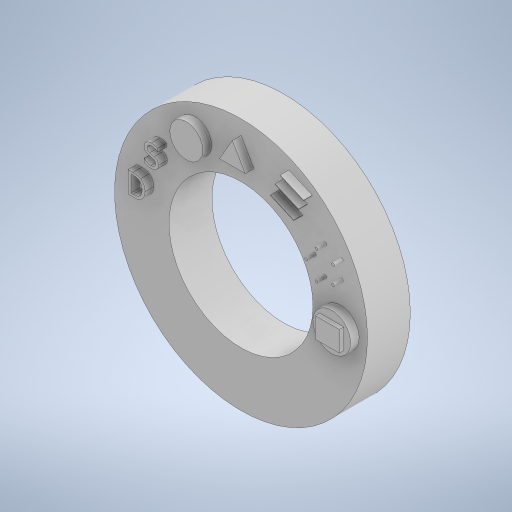
# Autodesk Inventor part: lab5CADfiguras
Saved by Autodesk Inventor 2023 (Build 270158000, 158)
## iProperties
Created: 2022-10-28
Part Number: lab5CADfiguras
Material: Generic
Document SubType Name: Modeling
Designer: jhair
Density: 1 g/cm^3
Appearance: Default
Author: jhair
Autodesk Inventor part; units mm, degrees
ref_plane "YZ Plane" through (0, 0, 0) normal (1, 0, 0) x (0, 1, 0)
ref_plane "XZ Plane" through (0, 0, 0) normal (0, 1, 0) x (-1, 0, 0)
ref_plane "XY Plane" through (0, 0, 0) normal (0, 0, 1) x (1, 0, 0)
sketch "Sketch1" plane through (0, 0, 0) normal (0, 0, 1) x (1, 0, 0)
  circle A0 centre (0, 0) radius 295
  circle A1 centre (0, 0) radius 168
  dimension "d0" = 590
  dimension "d1" = 336
  constraints: 2 centre point, 2 coincident
  measures "d0" diameter of A0
  measures "d1" diameter of A1
extrude "Extrusion1" add sketch "Sketch1" along normal blind 100
sketch "Sketch2" plane through (0, 0, 100) normal (0, 0, 1) x (1, 0, 0)
  line L0 (-208.7862, 161.4608) -> (-164.9221, 161.4608) construction
  line L1 (-164.9221, 161.4608) -> (-164.9221, 101.3592) construction
  line L2 (-164.9221, 101.3592) -> (-208.7862, 101.3592) construction
  line L3 (-208.7862, 101.3592) -> (-208.7862, 161.4608) construction
  line L4 (-248.2148, 80.7284) -> (-204.3506, 80.7284) construction
  line L5 (-204.3506, 80.7284) -> (-204.3506, 20.6268) construction
  line L6 (-204.3506, 20.6268) -> (-248.2148, 20.6268) construction
  line L7 (-248.2148, 20.6268) -> (-248.2148, 80.7284) construction
  spline S0 degree 2 poles (-189.783, 109.678) (-195.2125, 109.678) (-202.83, 111.947) (-206.193, 113.5678) knots 0 0 0 1 2 2 2
  line L8 (-206.193, 113.5678) -> (-206.193, 121.9146)
  line L9 (-206.193, 121.9146) -> (-205.7068, 121.9146)
  spline S1 degree 2 poles (-205.7068, 121.9146) (-202.4248, 118.8352) (-194.1185, 115.4316) (-190.2692, 115.4316) knots 0 0 0 1 2 2 2
  spline S2 degree 2 poles (-190.2692, 115.4316) (-184.7587, 115.4316) (-179.1266, 120.0102) (-179.1266, 123.7785) knots 0 0 0 1 2 2 2
  spline S3 degree 2 poles (-179.1266, 123.7785) (-179.1266, 126.7768) (-182.0845, 130.5046) (-185.2854, 131.4365) knots 0 0 0 1 2 2 2
  spline S4 degree 2 poles (-185.2854, 131.4365) (-187.595, 132.0848) (-191.4443, 132.9762) (-194.3211, 133.7055) knots 0 0 0 1 2 2 2
  spline S5 degree 2 poles (-194.3211, 133.7055) (-196.9143, 134.3943) (-201.0067, 136.4608) (-202.5869, 138.1221) knots 0 0 0 1 2 2 2
  spline S6 degree 2 poles (-202.5869, 138.1221) (-204.1266, 139.7833) (-205.8284, 144.2404) (-205.8284, 147.1577) knots 0 0 0 1 2 2 2
  spline S7 degree 2 poles (-205.8284, 147.1577) (-205.8284, 153.2355) (-196.347, 161.4608) (-189.0131, 161.4608) knots 0 0 0 1 2 2 2
  spline S8 degree 2 poles (-189.0131, 161.4608) (-184.7992, 161.4608) (-177.3438, 159.7995) (-174.1428, 158.2193) knots 0 0 0 1 2 2 2
  line L10 (-174.1428, 158.2193) -> (-174.1428, 150.2776)
  line L11 (-174.1428, 150.2776) -> (-174.629, 150.2776)
  spline S9 degree 2 poles (-174.629, 150.2776) (-177.0196, 152.4657) (-184.4751, 155.7071) (-188.5674, 155.7071) knots 0 0 0 1 2 2 2
  spline S10 degree 2 poles (-188.5674, 155.7071) (-193.1866, 155.7071) (-198.8997, 151.3717) (-198.8997, 147.8465) knots 0 0 0 1 2 2 2
  spline S11 degree 2 poles (-198.8997, 147.8465) (-198.8997, 144.6861) (-195.5366, 140.9178) (-192.3762, 140.067) knots 0 0 0 1 2 2 2
  spline S12 degree 2 poles (-192.3762, 140.067) (-190.2692, 139.4997) (-184.1509, 138.041) (-182.125, 137.4332) knots 0 0 0 1 2 2 2
  spline S13 degree 2 poles (-182.125, 137.4332) (-176.9791, 135.853) (-172.1979, 129.4916) (-172.1979, 124.8319) knots 0 0 0 1 2 2 2
  spline S14 degree 2 poles (-172.1979, 124.8319) (-172.1979, 121.8741) (-174.5885, 116.2015) (-176.736, 114.2161) knots 0 0 0 1 2 2 2
  spline S15 degree 2 poles (-176.736, 114.2161) (-179.1266, 112.0281) (-185.2044, 109.678) (-189.783, 109.678) knots 0 0 0 1 2 2 2
  spline S16 degree 2 poles (-203.7253, 55.6879) (-203.7253, 48.8402) (-209.2764, 37.8192) (-213.936, 34.7397) knots 0 0 0 1 2 2 2
  spline S17 degree 2 poles (-213.936, 34.7397) (-217.7448, 32.3491) (-225.5648, 30.7284) (-231.6426, 30.7284) knots 0 0 0 1 2 2 2
  line L12 (-231.6426, 30.7284) -> (-243.1499, 30.7284)
  line L13 (-243.1499, 30.7284) -> (-243.1499, 80.7284)
  line L14 (-243.1499, 80.7284) -> (-231.7642, 80.7284)
  spline S18 degree 2 poles (-231.7642, 80.7284) (-224.714, 80.7284) (-216.6913, 78.6214) (-213.855, 76.7576) knots 0 0 0 1 2 2 2
  spline S19 degree 2 poles (-213.855, 76.7576) (-209.0332, 73.5566) (-203.7253, 62.9812) (-203.7253, 55.6879) knots 0 0 0 1 2 2 2
  spline S20 degree 2 poles (-210.654, 55.7689) (-210.654, 61.5226) (-214.4627, 69.6668) (-218.231, 71.9764) knots 0 0 0 1 2 2 2
  spline S21 degree 2 poles (-218.231, 71.9764) (-220.9052, 73.5566) (-226.9425, 74.9748) (-231.4401, 74.9748) knots 0 0 0 1 2 2 2
  line L15 (-231.4401, 74.9748) -> (-236.5049, 74.9748)
  line L16 (-236.5049, 74.9748) -> (-236.5049, 36.482)
  line L17 (-236.5049, 36.482) -> (-231.4401, 36.482)
  spline S22 degree 2 poles (-231.4401, 36.482) (-227.0235, 36.482) (-220.3379, 37.9002) (-217.6232, 39.8046) knots 0 0 0 1 2 2 2
  spline S23 degree 2 poles (-217.6232, 39.8046) (-214.1386, 42.1547) (-210.654, 49.9342) (-210.654, 55.7689) knots 0 0 0 1 2 2 2
  point P0 (0, 0)
  constraints: 4 other
extrude "Extrusion2" add sketch "Sketch2" along normal blind 20
sketch "Sketch3" plane through (0, 0, 100) normal (0, 0, 1) x (1, 0, 0)
  circle A0 centre (-107.4544, 206.725) radius 38.7006
  line L0 (0, 260.9541) -> (30, 208.9926)
  line L1 (0, 260.9541) -> (60, 260.9541) construction
  line L2 (30, 208.9926) -> (-30, 208.9926)
  line L3 (-30, 208.9926) -> (0, 260.9541)
  line L4 (99.1241, 221.6176) -> (153.8823, 198.1595)
  line L5 (153.8823, 198.1595) -> (154.5516, 199.7218)
  line L6 (154.5516, 199.7218) -> (99.7934, 223.1799)
  line L7 (99.7934, 223.1799) -> (99.1241, 221.6176)
  line L8 (99.1241, 221.6176) -> (154.5516, 199.7218) construction
  line L9 (153.8823, 198.1595) -> (99.7934, 223.1799) construction
  line L10 (88.1405, 193.8335) -> (142.8987, 170.3754)
  line L11 (142.8987, 170.3754) -> (143.568, 171.9378)
  line L12 (143.568, 171.9378) -> (88.8098, 195.3958)
  line L13 (88.8098, 195.3958) -> (88.1405, 193.8335)
  line L14 (88.1405, 193.8335) -> (143.568, 171.9378) construction
  line L15 (142.8987, 170.3754) -> (88.8098, 195.3958) construction
  line L16 (110.8556, 245.3816) -> (165.6138, 221.9235)
  line L17 (165.6138, 221.9235) -> (166.2831, 223.4858)
  line L18 (166.2831, 223.4858) -> (111.5249, 246.9439)
  line L19 (111.5249, 246.9439) -> (110.8556, 245.3816)
  circle A1 centre (206.6962, 106.977) radius 34.8144
  circle A2 centre (171.8818, 106.977) radius 3.4311
  circle A3 centre (195.938, 73.8666) radius 3.4311
  circle A4 centre (234.8616, 86.5136) radius 3.4311
  circle A5 centre (234.8616, 127.4404) radius 3.4311
  circle A6 centre (195.938, 140.0875) radius 3.4311
  circle A7 centre (231.7388, -10.0458) radius 44.0014
  line L20 (199.303, 19.687) -> (264.1746, 19.687)
  line L21 (264.1746, 19.687) -> (264.1746, -39.7787)
  line L22 (264.1746, -39.7787) -> (199.303, -39.7787)
  line L23 (199.303, -39.7787) -> (199.303, 19.687)
  line L24 (199.303, 19.687) -> (264.1746, -39.7787) construction
  line L25 (264.1746, 19.687) -> (199.303, -39.7787) construction
  point P0 (0, 0)
  point P1 (126.8379, 210.6697)
  point P2 (115.8542, 182.8856)
  dimension "d6" = 60
  dimension "d7" = 60
  dimension "d8" = 60
  dimension "d9" = 60
  dimension "d12" = 360
  constraints: 52 end point, 8 parallel, 6 centre point, 6 midpoint, 4 perpendicular, 3 horizontal, 1 equal length, 1 horizontal alignment, 16 other
  measures "d6" distance of L0.start L0.end
  measures "d7" angle of L0 L1
  measures "d8" distance of L0.end L2.end
  measures "d9" angle of L0 L2
extrude "Extrusion3" add sketch "Sketch3" along normal blind 20 contours A0 | L0 L2 L3 | L7 L6 L5 L4 | L13 L12 L11 L10 | L19 L18 L17 L16 | A5 A1 | A1 A5 | A4 A1 | A1 A4 | A6 A1 | A1 A6 | A3 A1 | A1 A3 | A2 A1 | A1 A2 | A7 L21 | L20 A7 | L21 L22 L23 L20 | A7 L22 | L23 A7
sketch "Sketch4" plane through (231.7388, -10.0458, 120) normal (0, 0, 1) x (1, 0, 0)
  line L0 (-27.8414, 23.9777) -> (27.8414, 23.9777)
  line L1 (27.8414, 23.9777) -> (27.8414, -23.9777)
  line L2 (27.8414, -23.9777) -> (-27.8414, -23.9777)
  line L3 (-27.8414, -23.9777) -> (-27.8414, 23.9777)
  line L4 (-27.8414, 23.9777) -> (27.8414, -23.9777) construction
  line L5 (27.8414, 23.9777) -> (-27.8414, -23.9777) construction
  point P0 (-231.7388, 10.0458)
  point P1 (0, 0)
  constraints: 12 end point, 2 midpoint, 2 parallel, 1 horizontal, 1 perpendicular
extrude "Extrusion4" add sketch "Sketch4" along normal blind 10
body "Solid1"
